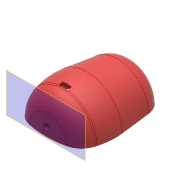
# Autodesk Inventor part: mask_back
Saved by Autodesk Inventor 2017 (Build 210142000, 142)
## iProperties
Created: 2018-06-30
Part Number: mask_back
Material: Generic
Document SubType Name: Modeling
Designer: mfans
Density: 1 g/cm^3
Appearance: Smooth - Red
Author: mfans
Autodesk Inventor part; units mm, degrees
ref_plane "YZ Plane" through (0, 0, 0) normal (1, 0, 0) x (0, 1, 0)
ref_plane "XY Plane" through (0, 0, 0) normal (0, 0, 1) x (1, 0, 0)
sketch "Sketch1" plane through (0, 0, 0) normal (0, 0, 1) x (1, 0, 0)
  line L0 (0, 0) -> (40, 0)
  arc A0 (0, -9.4427) -> (40, 0) centre (0, 80) ccw
  line L1 (40, 0) -> (30, 80)
  line L2 (30, 80) -> (0, 80)
  line L3 (0, 80) -> (0, -9.4427)
  dimension "d0" = 40
  dimension "d1" = 80
  dimension "d2" = 30
  constraints: 8 end point, 2 horizontal, 2 point on circle, 1 centre point, 1 perpendicular
  measures "d0" distance of L0.start L0.end
  measures "d1" distance of L0.start L2.end
  measures "d2" distance of L1.end L2.end
revolve "Revolution1" add sketch "Sketch1" angle 360 about axis through (0, 80, 0) along (0, -1, 0)
fillet "Fillet1" radius 20 1 edges at (-30, 80, 0)
chamfer "Chamfer1" distance 10 distance2 20 1 edges at (-40, 0, 0) measured on face at (-39.5522, -0.2224, 0)
fillet "Fillet2" radius 20 1 edges at (-30.8197, -3.9651, 0)
fillet "Fillet3" radius 60 1 edges at (-37.5193, 19.8456, 0)
sketch "Sketch2" plane through (0, 0, 0) normal (0, 0, 1) x (1, 0, 0)
  line L0 (-41.0234, 89.8189) -> (46.5058, 89.8189)
  line L1 (46.5058, 89.8189) -> (46.5058, -16.9931)
  line L2 (46.5058, -16.9931) -> (-41.0234, -16.9931)
  line L3 (-41.0234, -16.9931) -> (-41.0234, 89.8189)
  point P0 (0, 0)
  constraints: 8 end point, 2 parallel, 1 horizontal, 1 perpendicular
extrude "Extrusion1" cut sketch "Sketch2" against normal through all
shell "Shell1" thickness 4 removed faces 1 at (0, 18.1003, 0)
sketch "Sketch4" plane through (0, 0, 0) normal (0, 0, 1) x (1, 0, 0)
  line L0 (6, 0) -> (-6, 0)
  line L1 (-6, 0) -> (-6, -7.9457)
  line L2 (-6, -7.9457) -> (6, -7.9457)
  line L3 (6, -7.9457) -> (6, 0)
  point P0 (0, 0)
  dimension "d32" = 6
  dimension "d33" = 12
  constraints: 8 end point, 2 parallel, 1 horizontal, 1 perpendicular
  measures "d32" distance from line of L3 point (0, 0)
  measures "d33" distance of L0.start L0.end
extrude "Extrusion3" add sketch "Sketch4" along normal blind 14
sketch "Sketch5" plane through (-6, 0, 0) normal (0, 1, 0) x (1, 0, 0)
  line L0 (10, 12) -> (2, 12)
  line L1 (2, 12) -> (2, -12)
  line L2 (2, -12) -> (10, -12)
  line L3 (10, -12) -> (10, 12)
  line L4 (10, 12) -> (2, -12) construction
  line L5 (2, 12) -> (10, -12) construction
  point P0 (6, 0)
  dimension "d36" = 8
  dimension "d37" = 24
  constraints: 12 end point, 2 midpoint, 2 parallel, 1 horizontal, 1 perpendicular
  measures "d36" distance of L0.start L0.end
  measures "d37" distance of L0.end L1.end
extrude "Extrusion4" cut sketch "Sketch5" against normal blind 4
sketch "Sketch6" plane through (-6, -4, 0) normal (0, 1, 0) x (1, 0, 0)
  line L0 (2, 0) -> (10, 0) projected
  line L1 (2, -12) -> (2, 0) projected
  line L2 (10, -12) -> (2, -12) projected
  line L3 (10, 0) -> (10, -12) projected
  point P0 (6, 0)
  point P1 (6, -8)
  dimension "d40" = 8
  measures "d40" distance from line of L0 point (6, -8)
hole "Hole1" at (0, -4, 8) direction (0, -1, 0) diameter 3.5 end through all
ref_plane "Work Plane1" through (0, -9.5, 0) normal (0, 1, 0) x (-1, 0, 0)
sketch "Sketch7" plane through (0, -9.5, 0) normal (0, 1, 0) x (-1, 0, 0)
  spline S0 degree 5 poles (0, 9.75) (0.5302, 9.75) (1.061, 9.5496) (1.4864, 9.1462) (1.7161, 8.6301) (1.7803, 7.5328) (1.5832, 6.9485) (1.1379, 6.4793) (0.5686, 6.25) (-0.5686, 6.25) (-1.1379, 6.4793) (-1.5832, 6.9485) (-1.7803, 7.5328) (-1.7161, 8.6301) (-1.4864, 9.1462) (-1.061, 9.5496) (-0.5301, 9.75) (0, 9.75) knots 0 0 0 0 0 0 0.24055 0.24055 0.24055 0.24055 0.499999 0.499999 0.499999 0.499999 0.759449 0.759449 0.759449 0.759449 1 1 1 1 1 1 projected
  circle A0 centre (0, 8) radius 3
  point P0 (0, 0)
  dimension "d49" = 6
  constraints: 1 centre point, 1 other
  measures "d49" diameter of A0
extrude "Extrusion5" cut sketch "Sketch7" along normal blind 4
fillet "Fillet4" radius 2 2 edges at (-4, -2, 12) (4, -2, 12)
sketch "Sketch8" plane through (0, 0, 0) normal (0, 0, 1) x (1, 0, 0)
  line L0 (-10, 7) -> (10, 7)
  line L1 (10, 7) -> (10, 13)
  line L2 (10, 13) -> (-10, 13)
  line L3 (-10, 13) -> (-10, 7)
  line L4 (-10, 7) -> (10, 13) construction
  line L5 (10, 7) -> (-10, 13) construction
  point P0 (0, 0)
  point P1 (0, 10)
  dimension "d53" = 20
  dimension "d54" = 6
  dimension "d55" = 10
  constraints: 12 end point, 2 midpoint, 2 parallel, 1 horizontal, 1 perpendicular
  measures "d53" distance of L1.end L2.end
  measures "d54" distance of L2.end L0.start
  measures "d55" distance of point (0, 0) point (0, 10)
extrude "Extrusion6" cut sketch "Sketch8" along normal blind 32
sketch "Sketch9" plane through (0, 0, 32) normal (0, 0, -1) x (-1, 0, 0)
  line L0 (10, 7) -> (-10, 7) projected
  line L1 (10, 13) -> (10, 7) projected
  line L2 (-10, 13) -> (10, 13) projected
  line L3 (-10, 7) -> (-10, 13) projected
  line L4 (4.5, 8) -> (-4.5, 8)
  line L5 (-4.5, 8) -> (-4.5, 12)
  line L6 (-4.5, 12) -> (4.5, 12)
  line L7 (4.5, 12) -> (4.5, 8)
  line L8 (4.5, 8) -> (-4.5, 12) construction
  line L9 (-4.5, 8) -> (4.5, 12) construction
  point P0 (0, 0)
  point P1 (0, 10)
  dimension "d58" = 4
  dimension "d59" = 1
  dimension "d60" = 10
  dimension "d61" = 9
  constraints: 12 end point, 2 midpoint, 2 parallel, 1 horizontal, 1 perpendicular
  measures "d58" distance of L6.end L4.start
  measures "d59" distance between parallel lines of L0 L4
  measures "d60" distance from line of L3 point (0, 10)
  measures "d61" distance of L4.start L4.end
extrude "Extrusion7" cut sketch "Sketch9" against normal through all contours L4 L5 L6 L7
body "Solid1"
